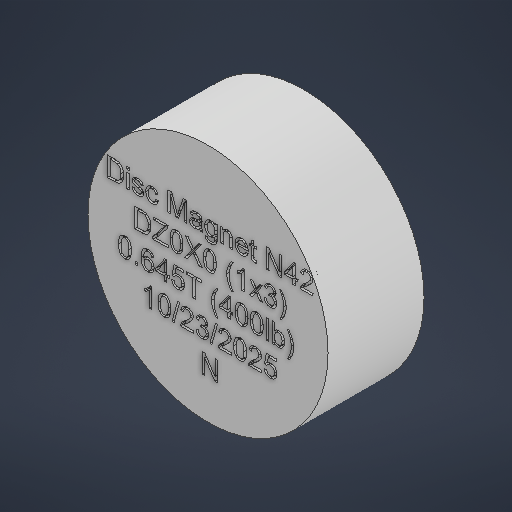
# Autodesk Inventor part: Sample_Magnet
Saved by Autodesk Inventor 2026.1 (Build 301233000, 233)
## iProperties
Created: 2025-10-23
Part Number: Sample_Magnet
Material: Generic
Document SubType Name: Modeling
Designer: usman
Density: 1 g/cm^3
Appearance: Default
Author: usman
Autodesk Inventor part; units mm, degrees
(part 1 of 2)
ref_plane "YZ Plane" through (0, 0, 0) normal (1, 0, 0) x (0, 1, 0)
ref_plane "XZ Plane" through (0, 0, 0) normal (0, 1, 0) x (-1, 0, 0)
ref_plane "XY Plane" through (0, 0, 0) normal (0, 0, 1) x (1, 0, 0)
sketch "Sketch1" plane through (0, 0, 0) normal (0, 0, 1) x (1, 0, 0)
  circle A0 centre (0, 0) radius 37.5
  dimension "d0" = 75
  constraints: 1 centre point, 1 coincident
  measures "d0" diameter of A0
extrude "Extrusion1" add sketch "Sketch1" along normal blind 30
sketch "Sketch2" plane through (0, 0, 30) normal (0, 0, 1) x (1, 0, 0)
  line L0 (-31.7477, 18.3387) -> (32.9347, 18.3387) construction
  line L1 (32.9347, 18.3387) -> (32.9347, -24.5034) construction
  line L2 (32.9347, -24.5034) -> (-31.7477, -24.5034) construction
  line L3 (-31.7477, -24.5034) -> (-31.7477, 18.3387) construction
  line L4 (-31.4082, 13.0446) -> (-31.4082, 19.1406)
  line L5 (-31.4082, 19.1406) -> (-29.308, 19.1406)
  spline S0 degree 2 poles (-29.308, 19.1406) (-28.5972, 19.1406) (-28.2208, 19.0523) knots 0 0 0 1 1 1
  spline S1 degree 2 poles (-28.2208, 19.0523) (-27.6958, 18.9315) (-27.3287, 18.6156) knots 0 0 0 1 1 1
  spline S2 degree 2 poles (-27.3287, 18.6156) (-26.8455, 18.2113) (-26.3669, 16.9429) (-26.3669, 16.1251) knots 0 0 0 1 2 2 2
  spline S3 degree 2 poles (-26.3669, 16.1251) (-26.3669, 15.4328) (-26.6922, 14.3595) (-27.1986, 13.6579) (-27.8026, 13.2537) (-28.6529, 13.0446) (-29.2058, 13.0446) knots 0 0 0 1 2 3 4 5 5 5
  line L6 (-29.2058, 13.0446) -> (-31.4082, 13.0446)
  line L7 (-30.5997, 13.7648) -> (-29.2988, 13.7648)
  spline S4 degree 2 poles (-29.2988, 13.7648) (-28.6947, 13.7648) (-28.0071, 13.9878) (-27.8073, 14.1922) knots 0 0 0 1 2 2 2
  spline S5 degree 2 poles (-27.8073, 14.1922) (-27.5192, 14.4803) (-27.1986, 15.4468) (-27.1986, 16.1391) knots 0 0 0 1 2 2 2
  spline S6 degree 2 poles (-27.1986, 16.1391) (-27.1986, 17.0962) (-27.8259, 18.123) (-28.2766, 18.295) knots 0 0 0 1 2 2 2
  spline S7 degree 2 poles (-28.2766, 18.295) (-28.6018, 18.4204) (-29.3173, 18.4204) knots 0 0 0 1 1 1
  line L8 (-29.3173, 18.4204) -> (-30.5997, 18.4204)
  line L9 (-30.5997, 18.4204) -> (-30.5997, 13.7648)
  line L10 (-25.3447, 13.0446) -> (-25.3447, 17.4633)
  line L11 (-25.3447, 17.4633) -> (-24.5967, 17.4633)
  line L12 (-24.5967, 17.4633) -> (-24.5967, 13.0446)
  line L13 (-24.5967, 13.0446) -> (-25.3447, 13.0446)
  line L14 (-25.3447, 18.281) -> (-25.3447, 19.1406)
  line L15 (-25.3447, 19.1406) -> (-24.5967, 19.1406)
  line L16 (-24.5967, 19.1406) -> (-24.5967, 18.281)
  line L17 (-24.5967, 18.281) -> (-25.3447, 18.281)
  line L18 (-23.7603, 14.3642) -> (-23.0215, 14.4803)
  spline S8 degree 2 poles (-23.0215, 14.4803) (-22.9611, 14.0343) (-22.3896, 13.5603) (-21.8739, 13.5603) knots 0 0 0 1 2 2 2
  spline S9 degree 2 poles (-21.8739, 13.5603) (-21.3582, 13.5603) (-20.8563, 13.9832) (-20.8563, 14.2666) knots 0 0 0 1 2 2 2
  spline S10 degree 2 poles (-20.8563, 14.2666) (-20.8563, 14.5175) (-21.0794, 14.6662) knots 0 0 0 1 1 1
  spline S11 degree 2 poles (-21.0794, 14.6662) (-21.2327, 14.7637) (-21.846, 14.9171) knots 0 0 0 1 1 1
  spline S12 degree 2 poles (-21.846, 14.9171) (-22.6684, 15.1262) (-23.305, 15.4282) (-23.6349, 15.9671) (-23.6349, 16.2877) knots 0 0 0 1 2 3 3 3
  spline S13 degree 2 poles (-23.6349, 16.2877) (-23.6349, 16.5851) (-23.3654, 17.0869) (-23.1331, 17.2542) knots 0 0 0 1 2 2 2
  spline S14 degree 2 poles (-23.1331, 17.2542) (-22.9565, 17.3843) (-22.3525, 17.5608) (-22.004, 17.5608) knots 0 0 0 1 2 2 2
  spline S15 degree 2 poles (-22.004, 17.5608) (-21.4836, 17.5608) (-20.6984, 17.2588) (-20.322, 16.7477) (-20.2523, 16.3203) knots 0 0 0 1 2 3 3 3
  line L19 (-20.2523, 16.3203) -> (-20.9864, 16.2227)
  spline S16 degree 2 poles (-20.9864, 16.2227) (-21.0376, 16.5665) (-21.5161, 16.9475) (-21.9529, 16.9475) knots 0 0 0 1 2 2 2
  spline S17 degree 2 poles (-21.9529, 16.9475) (-22.4686, 16.9475) (-22.91, 16.6037) (-22.91, 16.376) knots 0 0 0 1 2 2 2
  spline S18 degree 2 poles (-22.91, 16.376) (-22.91, 16.232) (-22.8171, 16.1158) knots 0 0 0 1 1 1
  spline S19 degree 2 poles (-22.8171, 16.1158) (-22.7288, 15.995) (-22.529, 15.916) knots 0 0 0 1 1 1
  spline S20 degree 2 poles (-22.529, 15.916) (-22.4175, 15.8742) (-21.8693, 15.7209) knots 0 0 0 1 1 1
  spline S21 degree 2 poles (-21.8693, 15.7209) (-21.0747, 15.5118) (-20.4428, 15.2423) (-20.0851, 14.7266) (-20.0851, 14.3409) knots 0 0 0 1 2 3 3 3
  spline S22 degree 2 poles (-20.0851, 14.3409) (-20.0851, 13.9692) (-20.5218, 13.3094) (-21.3489, 12.947) (-21.8693, 12.947) knots 0 0 0 1 2 3 3 3
  spline S23 degree 2 poles (-21.8693, 12.947) (-22.7288, 12.947) (-23.6349, 13.6626) (-23.7603, 14.3642) knots 0 0 0 1 2 2 2
  line L20 (-16.3122, 14.6615) -> (-15.5781, 14.564)
  spline S24 degree 2 poles (-15.5781, 14.564) (-15.6989, 13.8066) (-16.6932, 12.947) (-17.4181, 12.947) knots 0 0 0 1 2 2 2
  spline S25 degree 2 poles (-17.4181, 12.947) (-18.3241, 12.947) (-19.4253, 14.1318) (-19.4253, 15.2377) knots 0 0 0 1 2 2 2
  spline S26 degree 2 poles (-19.4253, 15.2377) (-19.4253, 15.9532) (-18.9513, 17.0265) (-17.9803, 17.5608) (-17.4134, 17.5608) knots 0 0 0 1 2 3 3 3
  spline S27 degree 2 poles (-17.4134, 17.5608) (-16.6932, 17.5608) (-15.7779, 16.8314) (-15.6478, 16.1623) knots 0 0 0 1 2 2 2
  line L21 (-15.6478, 16.1623) -> (-16.3773, 16.0508)
  spline S28 degree 2 poles (-16.3773, 16.0508) (-16.4795, 16.4968) (-17.0092, 16.9475) (-17.3809, 16.9475) knots 0 0 0 1 2 2 2
  spline S29 degree 2 poles (-17.3809, 16.9475) (-17.9477, 16.9475) (-18.654, 16.1344) (-18.654, 15.2563) knots 0 0 0 1 2 2 2
  spline S30 degree 2 poles (-18.654, 15.2563) (-18.654, 14.3688) (-17.971, 13.5603) (-17.4227, 13.5603) knots 0 0 0 1 2 2 2
  spline S31 degree 2 poles (-17.4227, 13.5603) (-16.9813, 13.5603) (-16.3912, 14.0993) (-16.3122, 14.6615) knots 0 0 0 1 2 2 2
  line L22 (-12.5022, 13.0446) -> (-12.5022, 19.1406)
  line L23 (-12.5022, 19.1406) -> (-11.2895, 19.1406)
  line L24 (-11.2895, 19.1406) -> (-9.8445, 14.8241)
  spline S32 degree 2 poles (-9.8445, 14.8241) (-9.6447, 14.2201) (-9.5518, 13.9228) knots 0 0 0 1 1 1
  spline S33 degree 2 poles (-9.5518, 13.9228) (-9.4496, 14.2526) (-9.2266, 14.8985) knots 0 0 0 1 1 1
  line L25 (-9.2266, 14.8985) -> (-7.763, 19.1406)
  line L26 (-7.763, 19.1406) -> (-6.6804, 19.1406)
  line L27 (-6.6804, 19.1406) -> (-6.6804, 13.0446)
  line L28 (-6.6804, 13.0446) -> (-7.4563, 13.0446)
  line L29 (-7.4563, 13.0446) -> (-7.4563, 18.1463)
  line L30 (-7.4563, 18.1463) -> (-9.2358, 13.0446)
  line L31 (-9.2358, 13.0446) -> (-9.9607, 13.0446)
  line L32 (-9.9607, 13.0446) -> (-11.7263, 18.2346)
  line L33 (-11.7263, 18.2346) -> (-11.7263, 13.0446)
  line L34 (-11.7263, 13.0446) -> (-12.5022, 13.0446)
  spline S34 degree 2 poles (-2.5962, 13.5882) (-3.0144, 13.2351) (-3.781, 12.947) (-4.2224, 12.947) knots 0 0 0 1 2 2 2
  spline S35 degree 2 poles (-4.2224, 12.947) (-4.9519, 12.947) (-5.7325, 13.6579) (-5.7325, 14.2108) knots 0 0 0 1 2 2 2
  spline S36 degree 2 poles (-5.7325, 14.2108) (-5.7325, 14.5361) (-5.4351, 15.0704) (-4.9612, 15.3956) (-4.6592, 15.4746) knots 0 0 0 1 2 3 3 3
  spline S37 degree 2 poles (-4.6592, 15.4746) (-4.4408, 15.535) (-3.9948, 15.5908) knots 0 0 0 1 1 1
  spline S38 degree 2 poles (-3.9948, 15.5908) (-3.0887, 15.6977) (-2.6613, 15.8463) knots 0 0 0 1 1 1
  spline S39 degree 2 poles (-2.6613, 15.8463) (-2.6566, 15.9997) (-2.6566, 16.0415) knots 0 0 0 1 1 1
  spline S40 degree 2 poles (-2.6566, 16.0415) (-2.6566, 16.5015) (-2.8704, 16.6873) knots 0 0 0 1 1 1
  spline S41 degree 2 poles (-2.8704, 16.6873) (-3.1538, 16.9429) (-3.7206, 16.9429) knots 0 0 0 1 1 1
  spline S42 degree 2 poles (-3.7206, 16.9429) (-4.2457, 16.9429) (-4.7475, 16.5712) (-4.8683, 16.1019) knots 0 0 0 1 2 2 2
  line L35 (-4.8683, 16.1019) -> (-5.6024, 16.1995)
  spline S43 degree 2 poles (-5.6024, 16.1995) (-5.5048, 16.6687) (-5.0448, 17.2495) (-4.1806, 17.5608) (-3.6138, 17.5608) knots 0 0 0 1 2 3 3 3
  spline S44 degree 2 poles (-3.6138, 17.5608) (-3.0469, 17.5608) (-2.3407, 17.296) (-2.0061, 16.8918) (-1.9411, 16.5851) knots 0 0 0 1 2 3 3 3
  spline S45 degree 2 poles (-1.9411, 16.5851) (-1.9039, 16.39) (-1.9039, 15.8928) knots 0 0 0 1 1 1
  line L36 (-1.9039, 15.8928) -> (-1.9039, 14.8938)
  spline S46 degree 2 poles (-1.9039, 14.8938) (-1.9039, 13.8531) (-1.8063, 13.3001) (-1.667, 13.0446) knots 0 0 0 1 2 2 2
  line L37 (-1.667, 13.0446) -> (-2.4475, 13.0446)
  spline S47 degree 2 poles (-2.4475, 13.0446) (-2.5637, 13.2769) (-2.5962, 13.5882) knots 0 0 0 1 1 1
  spline S48 degree 2 poles (-2.6566, 15.2609) (-3.0655, 15.0936) (-3.8786, 14.9775) knots 0 0 0 1 1 1
  spline S49 degree 2 poles (-3.8786, 14.9775) (-4.3433, 14.9124) (-4.7243, 14.7452) (-4.9333, 14.4246) (-4.9333, 14.2294) knots 0 0 0 1 2 3 3 3
  spline S50 degree 2 poles (-4.9333, 14.2294) (-4.9333, 13.932) (-4.4826, 13.5325) (-4.0459, 13.5325) knots 0 0 0 1 2 2 2
  spline S51 degree 2 poles (-4.0459, 13.5325) (-3.6138, 13.5325) (-2.9401, 13.9088) (-2.7821, 14.2387) knots 0 0 0 1 2 2 2
  spline S52 degree 2 poles (-2.7821, 14.2387) (-2.6613, 14.4943) (-2.6613, 14.9868) knots 0 0 0 1 1 1
  line L38 (-2.6613, 14.9868) -> (-2.6566, 15.2609)
  line L39 (-0.8817, 12.6822) -> (-0.1523, 12.5753)
  spline S53 degree 2 poles (-0.1523, 12.5753) (-0.1058, 12.2361) (0.1033, 12.0828) knots 0 0 0 1 1 1
  spline S54 degree 2 poles (0.1033, 12.0828) (0.3821, 11.8737) (0.8653, 11.8737) knots 0 0 0 1 1 1
  spline S55 degree 2 poles (0.8653, 11.8737) (1.381, 11.8737) (1.9479, 12.2872) (2.0501, 12.6636) knots 0 0 0 1 2 2 2
  spline S56 degree 2 poles (2.0501, 12.6636) (2.1059, 12.8913) (2.1012, 13.6207) knots 0 0 0 1 1 1
  spline S57 degree 2 poles (2.1012, 13.6207) (1.6134, 13.0446) (0.8792, 13.0446) knots 0 0 0 1 1 1
  spline S58 degree 2 poles (0.8792, 13.0446) (-0.0314, 13.0446) (-1.0304, 14.3595) (-1.0304, 15.2795) knots 0 0 0 1 2 2 2
  spline S59 degree 2 poles (-1.0304, 15.2795) (-1.0304, 15.9114) (-0.5704, 16.98) (0.2984, 17.5608) (0.8839, 17.5608) knots 0 0 0 1 2 3 3 3
  spline S60 degree 2 poles (0.8839, 17.5608) (1.6645, 17.5608) (2.1709, 16.9289) knots 0 0 0 1 1 1
  line L40 (2.1709, 16.9289) -> (2.1709, 17.4633)
  line L41 (2.1709, 17.4633) -> (2.8632, 17.4633)
  line L42 (2.8632, 17.4633) -> (2.8632, 13.6486)
  spline S61 degree 2 poles (2.8632, 13.6486) (2.8632, 12.6171) (2.4451, 11.7529) (1.5344, 11.2558) (0.8653, 11.2558) knots 0 0 0 1 2 3 3 3
  spline S62 degree 2 poles (0.8653, 11.2558) (0.0754, 11.2558) (-0.8957, 11.9666) (-0.8817, 12.6822) knots 0 0 0 1 2 2 2
  spline S63 degree 2 poles (-0.2591, 15.3306) (-0.2591, 14.4617) (0.4332, 13.6626) (0.9489, 13.6626) knots 0 0 0 1 2 2 2
  spline S64 degree 2 poles (0.9489, 13.6626) (1.4647, 13.6626) (2.1616, 14.4571) (2.1616, 15.3074) knots 0 0 0 1 2 2 2
  spline S65 degree 2 poles (2.1616, 15.3074) (2.1616, 16.1205) (1.4461, 16.9429) (0.9396, 16.9429) knots 0 0 0 1 2 2 2
  spline S66 degree 2 poles (0.9396, 16.9429) (0.4378, 16.9429) (-0.2591, 16.1298) (-0.2591, 15.3306) knots 0 0 0 1 2 2 2
  line L43 (3.9923, 13.0446) -> (3.9923, 17.4633)
  line L44 (3.9923, 17.4633) -> (4.666, 17.4633)
  line L45 (4.666, 17.4633) -> (4.666, 16.836)
  spline S67 degree 2 poles (4.666, 16.836) (5.1539, 17.5608) (6.0692, 17.5608) knots 0 0 0 1 1 1
  spline S68 degree 2 poles (6.0692, 17.5608) (6.4688, 17.5608) (7.1379, 17.2728) (7.4724, 16.8081) (7.5374, 16.4875) knots 0 0 0 1 2 3 3 3
  spline S69 degree 2 poles (7.5374, 16.4875) (7.5793, 16.2785) (7.5793, 15.7581) knots 0 0 0 1 1 1
  line L46 (7.5793, 15.7581) -> (7.5793, 13.0446)
  line L47 (7.5793, 13.0446) -> (6.8312, 13.0446)
  line L48 (6.8312, 13.0446) -> (6.8312, 15.7302)
  spline S70 degree 2 poles (6.8312, 15.7302) (6.8312, 16.1855) (6.6546, 16.6409) (6.2132, 16.9104) (5.9112, 16.9104) knots 0 0 0 1 2 3 3 3
  spline S71 degree 2 poles (5.9112, 16.9104) (5.4327, 16.9104) (4.7403, 16.3017) (4.7403, 15.456) knots 0 0 0 1 2 2 2
  line L49 (4.7403, 15.456) -> (4.7403, 13.0446)
  line L50 (4.7403, 13.0446) -> (3.9923, 13.0446)
  line L51 (11.747, 14.471) -> (12.523, 14.3735)
  spline S72 degree 2 poles (12.523, 14.3735) (12.3371, 13.6951) (11.3474, 12.947) (10.5808, 12.947) knots 0 0 0 1 2 2 2
  spline S73 degree 2 poles (10.5808, 12.947) (9.6097, 12.947) (8.476, 14.1411) (8.476, 15.2144) knots 0 0 0 1 2 2 2
  spline S74 degree 2 poles (8.476, 15.2144) (8.476, 16.3296) (9.6237, 17.5608) (10.539, 17.5608) knots 0 0 0 1 2 2 2
  spline S75 degree 2 poles (10.539, 17.5608) (11.4218, 17.5608) (12.5462, 16.3528) (12.5462, 15.2609) knots 0 0 0 1 2 2 2
  spline S76 degree 2 poles (12.5462, 15.2609) (12.5462, 15.1959) (12.5416, 15.0611) knots 0 0 0 1 1 1
  line L52 (12.5416, 15.0611) -> (9.2473, 15.0611)
  spline S77 degree 2 poles (9.2473, 15.0611) (9.2891, 14.3316) (10.0279, 13.5603) (10.5808, 13.5603) knots 0 0 0 1 2 2 2
  spline S78 degree 2 poles (10.5808, 13.5603) (10.9943, 13.5603) (11.5751, 13.9971) (11.747, 14.471) knots 0 0 0 1 2 2 2
  line L53 (9.2891, 15.6744) -> (11.7563, 15.6744)
  spline S79 degree 2 poles (11.7563, 15.6744) (11.7052, 16.232) (11.4729, 16.5154) knots 0 0 0 1 1 1
  spline S80 degree 2 poles (11.4729, 16.5154) (11.1151, 16.9475) (10.5436, 16.9475) knots 0 0 0 1 1 1
  spline S81 degree 2 poles (10.5436, 16.9475) (10.0279, 16.9475) (9.3263, 16.2552) (9.2891, 15.6744) knots 0 0 0 1 2 2 2
  line L54 (15.0924, 13.7137) -> (15.1993, 13.0492)
  spline S82 degree 2 poles (15.1993, 13.0492) (14.8833, 12.9842) (14.6324, 12.9842) knots 0 0 0 1 1 1
  spline S83 degree 2 poles (14.6324, 12.9842) (14.2282, 12.9842) (13.7775, 13.2444) (13.5963, 13.6626) (13.5963, 14.3363) knots 0 0 0 1 2 3 3 3
  line L55 (13.5963, 14.3363) -> (13.5963, 16.8825)
  line L56 (13.5963, 16.8825) -> (13.0434, 16.8825)
  line L57 (13.0434, 16.8825) -> (13.0434, 17.4633)
  line L58 (13.0434, 17.4633) -> (13.5963, 17.4633)
  line L59 (13.5963, 17.4633) -> (13.5963, 18.5552)
  line L60 (13.5963, 18.5552) -> (14.3443, 19.0059)
  line L61 (14.3443, 19.0059) -> (14.3443, 17.4633)
  line L62 (14.3443, 17.4633) -> (15.0924, 17.4633)
  line L63 (15.0924, 17.4633) -> (15.0924, 16.8825)
  line L64 (15.0924, 16.8825) -> (14.3443, 16.8825)
  line L65 (14.3443, 16.8825) -> (14.3443, 14.2945)
  spline S84 degree 2 poles (14.3443, 14.2945) (14.3443, 13.9739) (14.4233, 13.788) (14.5999, 13.6811) (14.7672, 13.6811) knots 0 0 0 1 2 3 3 3
  spline S85 degree 2 poles (14.7672, 13.6811) (14.888, 13.6811) (15.0924, 13.7137) knots 0 0 0 1 1 1
  line L66 (18.2798, 13.0446) -> (18.2798, 19.1406)
  line L67 (18.2798, 19.1406) -> (19.1068, 19.1406)
  line L68 (19.1068, 19.1406) -> (22.3128, 14.3549)
  line L69 (22.3128, 14.3549) -> (22.3128, 19.1406)
  line L70 (22.3128, 19.1406) -> (23.0841, 19.1406)
  line L71 (23.0841, 19.1406) -> (23.0841, 13.0446)
  line L72 (23.0841, 13.0446) -> (22.2571, 13.0446)
  line L73 (22.2571, 13.0446) -> (19.0511, 17.8303)
  line L74 (19.0511, 17.8303) -> (19.0511, 13.0446)
  line L75 (19.0511, 13.0446) -> (18.2798, 13.0446)
  line L76 (26.5317, 13.0446) -> (26.5317, 14.5035)
  line L77 (26.5317, 14.5035) -> (23.8879, 14.5035)
  line L78 (23.8879, 14.5035) -> (23.8879, 15.1912)
  line L79 (23.8879, 15.1912) -> (26.6664, 19.1406)
  line L80 (26.6664, 19.1406) -> (27.2797, 19.1406)
  line L81 (27.2797, 19.1406) -> (27.2797, 15.1912)
  line L82 (27.2797, 15.1912) -> (28.1022, 15.1912)
  line L83 (28.1022, 15.1912) -> (28.1022, 14.5035)
  line L84 (28.1022, 14.5035) -> (27.2797, 14.5035)
  line L85 (27.2797, 14.5035) -> (27.2797, 13.0446)
  line L86 (27.2797, 13.0446) -> (26.5317, 13.0446)
  line L87 (26.5317, 15.1912) -> (26.5317, 17.9418)
  line L88 (26.5317, 17.9418) -> (24.622, 15.1912)
  line L89 (24.622, 15.1912) -> (26.5317, 15.1912)
  line L90 (32.7996, 13.7648) -> (32.7996, 13.0446)
  line L91 (32.7996, 13.0446) -> (28.7712, 13.0446)
  spline S86 degree 2 poles (28.7712, 13.0446) (28.7619, 13.3141) (28.8595, 13.565) knots 0 0 0 1 1 1
  spline S87 degree 2 poles (28.8595, 13.565) (29.0128, 13.9785) (29.6912, 14.773) (30.3324, 15.2981) knots 0 0 0 1 2 2 2
  spline S88 degree 2 poles (30.3324, 15.2981) (31.3221, 16.1158) (32.019, 17.0637) (32.019, 17.4911) knots 0 0 0 1 2 2 2
  spline S89 degree 2 poles (32.019, 17.4911) (32.019, 17.9372) (31.3825, 18.5459) (30.8714, 18.5459) knots 0 0 0 1 2 2 2
  spline S90 degree 2 poles (30.8714, 18.5459) (30.3324, 18.5459) (29.6866, 17.8954) (29.6819, 17.3239) knots 0 0 0 1 2 2 2
  line L92 (29.6819, 17.3239) -> (28.9106, 17.4029)
  spline S91 degree 2 poles (28.9106, 17.4029) (28.9896, 18.2624) (30.0211, 19.1638) (30.89, 19.1638) knots 0 0 0 1 2 2 2
  spline S92 degree 2 poles (30.89, 19.1638) (31.7681, 19.1638) (32.7903, 18.1927) (32.7903, 17.4726) knots 0 0 0 1 2 2 2
  spline S93 degree 2 poles (32.7903, 17.4726) (32.7903, 17.1055) (32.4929, 16.3993) (31.796, 15.6187) (30.9922, 14.9357) knots 0 0 0 1 2 3 3 3
  spline S94 degree 2 poles (30.9922, 14.9357) (30.3185, 14.3735) (29.9375, 13.9692) (29.812, 13.7648) knots 0 0 0 1 2 2 2
  line L93 (29.812, 13.7648) -> (32.7996, 13.7648)
  line L94 (-22.8868, 3.4513) -> (-22.8868, 9.5473)
  line L95 (-22.8868, 9.5473) -> (-20.7867, 9.5473)
  spline S95 degree 2 poles (-20.7867, 9.5473) (-20.0758, 9.5473) (-19.6994, 9.459) knots 0 0 0 1 1 1
  spline S96 degree 2 poles (-19.6994, 9.459) (-19.1744, 9.3382) (-18.8073, 9.0223) knots 0 0 0 1 1 1
  spline S97 degree 2 poles (-18.8073, 9.0223) (-18.3241, 8.618) (-17.8455, 7.3496) (-17.8455, 6.5318) knots 0 0 0 1 2 2 2
  spline S98 degree 2 poles (-17.8455, 6.5318) (-17.8455, 5.8395) (-18.1708, 4.7662) (-18.6772, 4.0646) (-19.2812, 3.6604) (-20.1315, 3.4513) (-20.6844, 3.4513) knots 0 0 0 1 2 3 4 5 5 5
  line L96 (-20.6844, 3.4513) -> (-22.8868, 3.4513)
  line L97 (-22.0783, 4.1715) -> (-20.7774, 4.1715)
  spline S99 degree 2 poles (-20.7774, 4.1715) (-20.1733, 4.1715) (-19.4857, 4.3945) (-19.2859, 4.599) knots 0 0 0 1 2 2 2
  spline S100 degree 2 poles (-19.2859, 4.599) (-18.9978, 4.887) (-18.6772, 5.8535) (-18.6772, 6.5458) knots 0 0 0 1 2 2 2
  spline S101 degree 2 poles (-18.6772, 6.5458) (-18.6772, 7.5029) (-19.3045, 8.5298) (-19.7552, 8.7017) knots 0 0 0 1 2 2 2
  spline S102 degree 2 poles (-19.7552, 8.7017) (-20.0804, 8.8271) (-20.7959, 8.8271) knots 0 0 0 1 1 1
  line L98 (-20.7959, 8.8271) -> (-22.0783, 8.8271)
  line L99 (-22.0783, 8.8271) -> (-22.0783, 4.1715)
  line L100 (-17.2229, 3.4513) -> (-17.2229, 4.1994)
  line L101 (-17.2229, 4.1994) -> (-14.0959, 8.1023)
  spline S103 degree 2 poles (-14.0959, 8.1023) (-13.7614, 8.5158) (-13.4594, 8.8271) knots 0 0 0 1 1 1
  line L102 (-13.4594, 8.8271) -> (-16.8698, 8.8271)
  line L103 (-16.8698, 8.8271) -> (-16.8698, 9.5473)
  line L104 (-16.8698, 9.5473) -> (-12.4976, 9.5473)
  line L105 (-12.4976, 9.5473) -> (-12.4976, 8.8271)
  line L106 (-12.4976, 8.8271) -> (-15.9266, 4.6036)
  line L107 (-15.9266, 4.6036) -> (-16.2936, 4.1715)
  line L108 (-16.2936, 4.1715) -> (-12.4, 4.1715)
  line L109 (-12.4, 4.1715) -> (-12.4, 3.4513)
  line L110 (-12.4, 3.4513) -> (-17.2229, 3.4513)
  spline S104 degree 2 poles (-11.8332, 6.4575) (-11.8332, 7.5401) (-11.3871, 8.8596) (-10.5136, 9.5705) (-9.8445, 9.5705) knots 0 0 0 1 2 3 3 3
  spline S105 degree 2 poles (-9.8445, 9.5705) (-9.3567, 9.5705) (-8.6132, 9.1756) (-8.1347, 8.4322) (-7.8605, 7.3635) (-7.8605, 6.4575) knots 0 0 0 1 2 3 4 4 4
  spline S106 degree 2 poles (-7.8605, 6.4575) (-7.8605, 5.3842) (-8.3019, 4.0646) (-9.1801, 3.3491) (-9.8445, 3.3491) knots 0 0 0 1 2 3 3 3
  spline S107 degree 2 poles (-9.8445, 3.3491) (-10.7273, 3.3491) (-11.2291, 3.9763) knots 0 0 0 1 1 1
  spline S108 degree 2 poles (-11.2291, 3.9763) (-11.8332, 4.743) (-11.8332, 6.4575) knots 0 0 0 1 1 1
  spline S109 degree 2 poles (-11.0619, 6.4575) (-11.0619, 4.9521) (-10.3603, 3.9624) (-9.8445, 3.9624) knots 0 0 0 1 2 2 2
  spline S110 degree 2 poles (-9.8445, 3.9624) (-9.3334, 3.9624) (-8.6318, 4.9567) (-8.6318, 6.4575) knots 0 0 0 1 2 2 2
  spline S111 degree 2 poles (-8.6318, 6.4575) (-8.6318, 7.9629) (-9.3334, 8.9526) (-9.8538, 8.9526) knots 0 0 0 1 2 2 2
  spline S112 degree 2 poles (-9.8538, 8.9526) (-10.3696, 8.9526) (-10.6762, 8.5158) knots 0 0 0 1 1 1
  spline S113 degree 2 poles (-10.6762, 8.5158) (-11.0619, 7.9583) (-11.0619, 6.4575) knots 0 0 0 1 1 1
  line L111 (-7.4145, 3.4513) -> (-5.0588, 6.6108)
  line L112 (-5.0588, 6.6108) -> (-7.1357, 9.5473)
  line L113 (-7.1357, 9.5473) -> (-6.1786, 9.5473)
  line L114 (-6.1786, 9.5473) -> (-5.0634, 7.9861)
  spline S114 degree 2 poles (-5.0634, 7.9861) (-4.715, 7.5029) (-4.5756, 7.2381) knots 0 0 0 1 1 1
  spline S115 degree 2 poles (-4.5756, 7.2381) (-4.3711, 7.5633) (-4.0877, 7.9257) knots 0 0 0 1 1 1
  line L115 (-4.0877, 7.9257) -> (-2.8704, 9.5473)
  line L116 (-2.8704, 9.5473) -> (-1.9922, 9.5473)
  line L117 (-1.9922, 9.5473) -> (-4.1063, 6.648)
  line L118 (-4.1063, 6.648) -> (-1.8249, 3.4513)
  line L119 (-1.8249, 3.4513) -> (-2.8146, 3.4513)
  line L120 (-2.8146, 3.4513) -> (-4.3572, 5.6258)
  spline S116 degree 2 poles (-4.3572, 5.6258) (-4.4873, 5.8116) (-4.6127, 6.0021) knots 0 0 0 1 1 1
  spline S117 degree 2 poles (-4.6127, 6.0021) (-4.8125, 5.6908) (-4.9008, 5.5654) knots 0 0 0 1 1 1
  line L121 (-4.9008, 5.5654) -> (-6.4434, 3.4513)
  line L122 (-6.4434, 3.4513) -> (-7.4145, 3.4513)
  spline S118 degree 2 poles (-1.4161, 6.4575) (-1.4161, 7.5401) (-0.97, 8.8596) (-0.0965, 9.5705) (0.5726, 9.5705) knots 0 0 0 1 2 3 3 3
  spline S119 degree 2 poles (0.5726, 9.5705) (1.0604, 9.5705) (1.8039, 9.1756) (2.2824, 8.4322) (2.5566, 7.3635) (2.5566, 6.4575) knots 0 0 0 1 2 3 4 4 4
  spline S120 degree 2 poles (2.5566, 6.4575) (2.5566, 5.3842) (2.1152, 4.0646) (1.237, 3.3491) (0.5726, 3.3491) knots 0 0 0 1 2 3 3 3
  spline S121 degree 2 poles (0.5726, 3.3491) (-0.3102, 3.3491) (-0.812, 3.9763) knots 0 0 0 1 1 1
  spline S122 degree 2 poles (-0.812, 3.9763) (-1.4161, 4.743) (-1.4161, 6.4575) knots 0 0 0 1 1 1
  spline S123 degree 2 poles (-0.6448, 6.4575) (-0.6448, 4.9521) (0.0568, 3.9624) (0.5726, 3.9624) knots 0 0 0 1 2 2 2
  spline S124 degree 2 poles (0.5726, 3.9624) (1.0837, 3.9624) (1.7853, 4.9567) (1.7853, 6.4575) knots 0 0 0 1 2 2 2
  spline S125 degree 2 poles (1.7853, 6.4575) (1.7853, 7.9629) (1.0837, 8.9526) (0.5633, 8.9526) knots 0 0 0 1 2 2 2
  spline S126 degree 2 poles (0.5633, 8.9526) (0.0475, 8.9526) (-0.2591, 8.5158) knots 0 0 0 1 1 1
  spline S127 degree 2 poles (-0.2591, 8.5158) (-0.6448, 7.9583) (-0.6448, 6.4575) knots 0 0 0 1 1 1
  spline S128 degree 2 poles (7.3237, 1.6578) (6.7058, 2.4384) (5.8462, 4.5339) (5.8462, 5.6583) knots 0 0 0 1 2 2 2
  spline S129 degree 2 poles (5.8462, 5.6583) (5.8462, 6.648) (6.1668, 7.554) knots 0 0 0 1 1 1
  spline S130 degree 2 poles (6.1668, 7.554) (6.5431, 8.6041) (7.3237, 9.6495) knots 0 0 0 1 1 1
  line L123 (7.3237, 9.6495) -> (7.858, 9.6495)
  spline S131 degree 2 poles (7.858, 9.6495) (7.3562, 8.7853) (7.1936, 8.4136) knots 0 0 0 1 1 1
  spline S132 degree 2 poles (7.1936, 8.4136) (6.9427, 7.8421) (6.794, 7.2148) knots 0 0 0 1 1 1
  spline S133 degree 2 poles (6.794, 7.2148) (6.6175, 6.4389) (6.6175, 5.6537) knots 0 0 0 1 1 1
  spline S134 degree 2 poles (6.6175, 5.6537) (6.6175, 3.6557) (7.858, 1.6578) knots 0 0 0 1 1 1
  line L124 (7.858, 1.6578) -> (7.3237, 1.6578)
  line L125 (11.3335, 3.4513) -> (10.5854, 3.4513)
  line L126 (10.5854, 3.4513) -> (10.5854, 8.2185)
  spline S135 degree 2 poles (10.5854, 8.2185) (10.316, 7.9629) (9.4378, 7.4472) (9.0893, 7.3171) knots 0 0 0 1 2 2 2
  line L127 (9.0893, 7.3171) -> (9.0893, 8.0419)
  spline S136 degree 2 poles (9.0893, 8.0419) (9.7166, 8.3346) (10.6551, 9.1756) (10.8503, 9.5705) knots 0 0 0 1 2 2 2
  line L128 (10.8503, 9.5705) -> (11.3335, 9.5705)
  line L129 (11.3335, 9.5705) -> (11.3335, 3.4513)
  line L130 (12.9597, 3.4513) -> (14.5767, 5.7373)
  line L131 (14.5767, 5.7373) -> (13.0805, 7.87)
  line L132 (13.0805, 7.87) -> (14.0098, 7.87)
  line L133 (14.0098, 7.87) -> (14.6975, 6.8338)
  spline S137 degree 2 poles (14.6975, 6.8338) (14.8926, 6.5411) (15.0088, 6.346) knots 0 0 0 1 1 1
  spline S138 degree 2 poles (15.0088, 6.346) (15.1946, 6.6062) (15.3433, 6.8199) knots 0 0 0 1 1 1
  line L134 (15.3433, 6.8199) -> (16.0867, 7.87)
  line L135 (16.0867, 7.87) -> (16.9881, 7.87)
  line L136 (16.9881, 7.87) -> (15.492, 5.7512)
  line L137 (15.492, 5.7512) -> (17.095, 3.4513)
  line L138 (17.095, 3.4513) -> (16.175, 3.4513)
  line L139 (16.175, 3.4513) -> (15.2643, 4.8173)
  line L140 (15.2643, 4.8173) -> (15.0506, 5.1519)
  line L141 (15.0506, 5.1519) -> (13.8658, 3.4513)
  line L142 (13.8658, 3.4513) -> (12.9597, 3.4513)
  line L143 (17.5178, 5.0682) -> (18.2658, 5.1658)
  spline S139 degree 2 poles (18.2658, 5.1658) (18.3959, 4.5293) (19.0139, 3.9671) (19.46, 3.9671) knots 0 0 0 1 2 2 2
  spline S140 degree 2 poles (19.46, 3.9671) (19.9896, 3.9671) (20.7145, 4.7012) (20.7145, 5.2401) knots 0 0 0 1 2 2 2
  spline S141 degree 2 poles (20.7145, 5.2401) (20.7145, 5.7559) (20.0408, 6.425) (19.5204, 6.425) knots 0 0 0 1 2 2 2
  spline S142 degree 2 poles (19.5204, 6.425) (19.3113, 6.425) (18.9953, 6.3413) knots 0 0 0 1 1 1
  line L144 (18.9953, 6.3413) -> (19.0743, 6.9965)
  spline S143 degree 2 poles (19.0743, 6.9965) (19.1533, 6.9872) (19.1951, 6.9872) knots 0 0 0 1 1 1
  spline S144 degree 2 poles (19.1951, 6.9872) (19.6737, 6.9872) (20.4403, 7.489) (20.4403, 8.0047) knots 0 0 0 1 2 2 2
  spline S145 degree 2 poles (20.4403, 8.0047) (20.4403, 8.4182) (19.8828, 8.9572) (19.4414, 8.9572) knots 0 0 0 1 2 2 2
  spline S146 degree 2 poles (19.4414, 8.9572) (19.0046, 8.9572) (18.4238, 8.409) (18.3402, 7.856) knots 0 0 0 1 2 2 2
  line L145 (18.3402, 7.856) -> (17.5921, 7.9908)
  spline S147 degree 2 poles (17.5921, 7.9908) (17.7315, 8.7435) (18.7026, 9.5705) (19.4274, 9.5705) knots 0 0 0 1 2 2 2
  spline S148 degree 2 poles (19.4274, 9.5705) (19.9246, 9.5705) (20.7656, 9.1431) (21.2116, 8.4043) (21.2116, 7.9908) knots 0 0 0 1 2 3 3 3
  spline S149 degree 2 poles (21.2116, 7.9908) (21.2116, 7.5958) (20.7888, 6.9454) (20.3706, 6.7549) knots 0 0 0 1 2 2 2
  spline S150 degree 2 poles (20.3706, 6.7549) (20.9143, 6.6294) (21.509, 5.8442) (21.509, 5.2541) knots 0 0 0 1 2 2 2
  spline S151 degree 2 poles (21.509, 5.2541) (21.509, 4.4596) (20.3428, 3.3491) (19.4553, 3.3491) knots 0 0 0 1 2 2 2
  spline S152 degree 2 poles (19.4553, 3.3491) (18.6515, 3.3491) (17.5921, 4.3062) (17.5178, 5.0682) knots 0 0 0 1 2 2 2
  line L146 (22.9447, 1.6578) -> (22.4104, 1.6578)
  spline S153 degree 2 poles (22.4104, 1.6578) (23.651, 3.6557) (23.651, 5.6537) knots 0 0 0 1 1 1
  spline S154 degree 2 poles (23.651, 5.6537) (23.651, 6.4343) (23.4744, 7.2056) knots 0 0 0 1 1 1
  spline S155 degree 2 poles (23.4744, 7.2056) (23.3304, 7.8282) (23.0795, 8.4043) knots 0 0 0 1 1 1
  spline S156 degree 2 poles (23.0795, 8.4043) (22.9168, 8.776) (22.4104, 9.6495) knots 0 0 0 1 1 1
  line L147 (22.4104, 9.6495) -> (22.9447, 9.6495)
  spline S157 degree 2 poles (22.9447, 9.6495) (23.7253, 8.6041) (24.1017, 7.554) knots 0 0 0 1 1 1
  spline S158 degree 2 poles (24.1017, 7.554) (24.4223, 6.648) (24.4223, 5.6583) knots 0 0 0 1 1 1
  spline S159 degree 2 poles (24.4223, 5.6583) (24.4223, 4.5339) (23.5627, 2.4384) (22.9447, 1.6578) knots 0 0 0 1 2 2 2
  spline S160 degree 2 poles (-27.9211, -3.1358) (-27.9211, -2.0532) (-27.4751, -0.7336) (-26.6015, -0.0228) (-25.9325, -0.0228) knots 0 0 0 1 2 3 3 3
  spline S161 degree 2 poles (-25.9325, -0.0228) (-25.4446, -0.0228) (-24.7012, -0.4177) (-24.2226, -1.1611) (-23.9485, -2.2298) (-23.9485, -3.1358) knots 0 0 0 1 2 3 4 4 4
  spline S162 degree 2 poles (-23.9485, -3.1358) (-23.9485, -4.2091) (-24.3899, -5.5287) (-25.268, -6.2442) (-25.9325, -6.2442) knots 0 0 0 1 2 3 3 3
  spline S163 degree 2 poles (-25.9325, -6.2442) (-26.8153, -6.2442) (-27.3171, -5.6169) knots 0 0 0 1 1 1
  spline S164 degree 2 poles (-27.3171, -5.6169) (-27.9211, -4.8503) (-27.9211, -3.1358) knots 0 0 0 1 1 1
  spline S165 degree 2 poles (-27.1498, -3.1358) (-27.1498, -4.6412) (-26.4482, -5.6309) (-25.9325, -5.6309) knots 0 0 0 1 2 2 2
  spline S166 degree 2 poles (-25.9325, -5.6309) (-25.4214, -5.6309) (-24.7198, -4.6366) (-24.7198, -3.1358) knots 0 0 0 1 2 2 2
  spline S167 degree 2 poles (-24.7198, -3.1358) (-24.7198, -1.6304) (-25.4214, -0.6407) (-25.9418, -0.6407) knots 0 0 0 1 2 2 2
  spline S168 degree 2 poles (-25.9418, -0.6407) (-26.4575, -0.6407) (-26.7642, -1.0775) knots 0 0 0 1 1 1
  spline S169 degree 2 poles (-26.7642, -1.0775) (-27.1498, -1.635) (-27.1498, -3.1358) knots 0 0 0 1 1 1
  line L148 (-22.7683, -6.142) -> (-22.7683, -5.2917)
  line L149 (-22.7683, -5.2917) -> (-21.918, -5.2917)
  line L150 (-21.918, -5.2917) -> (-21.918, -6.142)
  line L151 (-21.918, -6.142) -> (-22.7683, -6.142)
  line L152 (-16.9325, -1.5421) -> (-17.6759, -1.6025)
  spline S170 degree 2 poles (-17.6759, -1.6025) (-17.7781, -1.1611) (-17.9594, -0.9567) knots 0 0 0 1 1 1
  spline S171 degree 2 poles (-17.9594, -0.9567) (-18.266, -0.6361) (-18.7121, -0.6361) knots 0 0 0 1 1 1
  spline S172 degree 2 poles (-18.7121, -0.6361) (-19.0698, -0.6361) (-19.3393, -0.8359) knots 0 0 0 1 1 1
  spline S173 degree 2 poles (-19.3393, -0.8359) (-19.6924, -1.0914) (-20.1013, -2.0857) (-20.1106, -3.0011) knots 0 0 0 1 2 2 2
  spline S174 degree 2 poles (-20.1106, -3.0011) (-19.8411, -2.5875) (-19.0559, -2.1879) (-18.6284, -2.1879) knots 0 0 0 1 2 2 2
  spline S175 degree 2 poles (-18.6284, -2.1879) (-17.8804, -2.1879) (-16.8256, -3.2891) (-16.8256, -4.1626) knots 0 0 0 1 2 2 2
  spline S176 degree 2 poles (-16.8256, -4.1626) (-16.8256, -4.7341) (-17.3228, -5.7192) (-18.187, -6.2442) (-18.7353, -6.2442) knots 0 0 0 1 2 3 3 3
  spline S177 degree 2 poles (-18.7353, -6.2442) (-19.6739, -6.2442) (-20.854, -4.8689) (-20.854, -3.2891) knots 0 0 0 1 2 2 2
  spline S178 degree 2 poles (-20.854, -3.2891) (-20.854, -1.5235) (-20.1989, -0.7197) knots 0 0 0 1 1 1
  spline S179 degree 2 poles (-20.1989, -0.7197) (-19.632, -0.0228) (-18.6656, -0.0228) knots 0 0 0 1 1 1
  spline S180 degree 2 poles (-18.6656, -0.0228) (-17.9454, -0.0228) (-17.0254, -0.8312) (-16.9325, -1.5421) knots 0 0 0 1 2 2 2
  spline S181 degree 2 poles (-19.9945, -4.1673) (-19.9945, -4.5529) (-19.6646, -5.2592) (-19.0791, -5.6309) (-18.7539, -5.6309) knots 0 0 0 1 2 3 3 3
  spline S182 degree 2 poles (-18.7539, -5.6309) (-18.2753, -5.6309) (-17.5969, -4.8642) (-17.5969, -4.2091) knots 0 0 0 1 2 2 2
  spline S183 degree 2 poles (-17.5969, -4.2091) (-17.5969, -3.5772) (-18.266, -2.8477) (-18.7818, -2.8477) knots 0 0 0 1 2 2 2
  spline S184 degree 2 poles (-18.7818, -2.8477) (-19.2882, -2.8477) (-19.9945, -3.5772) (-19.9945, -4.1673) knots 0 0 0 1 2 2 2
  line L153 (-13.6894, -6.142) -> (-13.6894, -4.683)
  line L154 (-13.6894, -4.683) -> (-16.3331, -4.683)
  line L155 (-16.3331, -4.683) -> (-16.3331, -3.9954)
  line L156 (-16.3331, -3.9954) -> (-13.5546, -0.046)
  line L157 (-13.5546, -0.046) -> (-12.9413, -0.046)
  line L158 (-12.9413, -0.046) -> (-12.9413, -3.9954)
  line L159 (-12.9413, -3.9954) -> (-12.1189, -3.9954)
  line L160 (-12.1189, -3.9954) -> (-12.1189, -4.683)
  line L161 (-12.1189, -4.683) -> (-12.9413, -4.683)
  line L162 (-12.9413, -4.683) -> (-12.9413, -6.142)
  line L163 (-12.9413, -6.142) -> (-13.6894, -6.142)
  line L164 (-13.6894, -3.9954) -> (-13.6894, -1.2447)
  line L165 (-13.6894, -1.2447) -> (-15.599, -3.9954)
  line L166 (-15.599, -3.9954) -> (-13.6894, -3.9954)
  line L167 (-11.3523, -4.5436) -> (-10.567, -4.4786)
  spline S185 degree 2 poles (-10.567, -4.4786) (-10.4787, -5.0547) (-9.8468, -5.6309) (-9.3961, -5.6309) knots 0 0 0 1 2 2 2
  spline S186 degree 2 poles (-9.3961, -5.6309) (-8.8479, -5.6309) (-8.1045, -4.8131) (-8.1045, -4.1394) knots 0 0 0 1 2 2 2
  spline S187 degree 2 poles (-8.1045, -4.1394) (-8.1045, -3.4982) (-8.82, -2.7548) (-9.4054, -2.7548) knots 0 0 0 1 2 2 2
  spline S188 degree 2 poles (-9.4054, -2.7548) (-9.7679, -2.7548) (-10.3486, -3.0847) (-10.5159, -3.3495) knots 0 0 0 1 2 2 2
  line L168 (-10.5159, -3.3495) -> (-11.2175, -3.2566)
  line L169 (-11.2175, -3.2566) -> (-10.6274, -0.125)
  line L170 (-10.6274, -0.125) -> (-7.598, -0.125)
  line L171 (-7.598, -0.125) -> (-7.598, -0.8405)
  line L172 (-7.598, -0.8405) -> (-10.028, -0.8405)
  line L173 (-10.028, -0.8405) -> (-10.3579, -2.476)
  spline S189 degree 2 poles (-10.3579, -2.476) (-9.8097, -2.095) (-9.2056, -2.095) knots 0 0 0 1 1 1
  spline S190 degree 2 poles (-9.2056, -2.095) (-8.4065, -2.095) (-7.3099, -3.2008) (-7.3099, -4.0697) knots 0 0 0 1 2 2 2
  spline S191 degree 2 poles (-7.3099, -4.0697) (-7.3099, -4.9014) (-7.7932, -5.5054) knots 0 0 0 1 1 1
  spline S192 degree 2 poles (-7.7932, -5.5054) (-8.3786, -6.2442) (-9.3915, -6.2442) knots 0 0 0 1 1 1
  spline S193 degree 2 poles (-9.3915, -6.2442) (-10.2232, -6.2442) (-11.2779, -5.3149) (-11.3523, -4.5436) knots 0 0 0 1 2 2 2
  line L174 (-4.7637, -6.142) -> (-4.7637, -0.7662)
  line L175 (-4.7637, -0.7662) -> (-6.771, -0.7662)
  line L176 (-6.771, -0.7662) -> (-6.771, -0.046)
  line L177 (-6.771, -0.046) -> (-1.9388, -0.046)
  line L178 (-1.9388, -0.046) -> (-1.9388, -0.7662)
  line L179 (-1.9388, -0.7662) -> (-3.9553, -0.7662)
  line L180 (-3.9553, -0.7662) -> (-3.9553, -6.142)
  line L181 (-3.9553, -6.142) -> (-4.7637, -6.142)
  spline S194 degree 2 poles (2.5914, -7.9355) (1.9735, -7.1549) (1.1139, -5.0594) (1.1139, -3.935) knots 0 0 0 1 2 2 2
  spline S195 degree 2 poles (1.1139, -3.935) (1.1139, -2.9453) (1.4345, -2.0393) knots 0 0 0 1 1 1
  spline S196 degree 2 poles (1.4345, -2.0393) (1.8108, -0.9892) (2.5914, 0.0562) knots 0 0 0 1 1 1
  line L182 (2.5914, 0.0562) -> (3.1257, 0.0562)
  spline S197 degree 2 poles (3.1257, 0.0562) (2.6239, -0.808) (2.4613, -1.1797) knots 0 0 0 1 1 1
  spline S198 degree 2 poles (2.4613, -1.1797) (2.2104, -1.7512) (2.0617, -2.3784) knots 0 0 0 1 1 1
  spline S199 degree 2 poles (2.0617, -2.3784) (1.8852, -3.1544) (1.8852, -3.9396) knots 0 0 0 1 1 1
  spline S200 degree 2 poles (1.8852, -3.9396) (1.8852, -5.9375) (3.1257, -7.9355) knots 0 0 0 1 1 1
  line L183 (3.1257, -7.9355) -> (2.5914, -7.9355)
  line L184 (6.183, -6.142) -> (6.183, -4.683)
  line L185 (6.183, -4.683) -> (3.5393, -4.683)
  line L186 (3.5393, -4.683) -> (3.5393, -3.9954)
  line L187 (3.5393, -3.9954) -> (6.3178, -0.046)
  line L188 (6.3178, -0.046) -> (6.9311, -0.046)
  line L189 (6.9311, -0.046) -> (6.9311, -3.9954)
  line L190 (6.9311, -3.9954) -> (7.7535, -3.9954)
  line L191 (7.7535, -3.9954) -> (7.7535, -4.683)
  line L192 (7.7535, -4.683) -> (6.9311, -4.683)
  line L193 (6.9311, -4.683) -> (6.9311, -6.142)
  line L194 (6.9311, -6.142) -> (6.183, -6.142)
  line L195 (6.183, -3.9954) -> (6.183, -1.2447)
  line L196 (6.183, -1.2447) -> (4.2734, -3.9954)
  line L197 (4.2734, -3.9954) -> (6.183, -3.9954)
  spline S201 degree 2 poles (8.5201, -3.1358) (8.5201, -2.0532) (8.9662, -0.7336) (9.8397, -0.0228) (10.5088, -0.0228) knots 0 0 0 1 2 3 3 3
  spline S202 degree 2 poles (10.5088, -0.0228) (10.9966, -0.0228) (11.7401, -0.4177) (12.2186, -1.1611) (12.4928, -2.2298) (12.4928, -3.1358) knots 0 0 0 1 2 3 4 4 4
  spline S203 degree 2 poles (12.4928, -3.1358) (12.4928, -4.2091) (12.0514, -5.5287) (11.1732, -6.2442) (10.5088, -6.2442) knots 0 0 0 1 2 3 3 3
  spline S204 degree 2 poles (10.5088, -6.2442) (9.626, -6.2442) (9.1242, -5.6169) knots 0 0 0 1 1 1
  spline S205 degree 2 poles (9.1242, -5.6169) (8.5201, -4.8503) (8.5201, -3.1358) knots 0 0 0 1 1 1
  spline S206 degree 2 poles (9.2914, -3.1358) (9.2914, -4.6412) (9.993, -5.6309) (10.5088, -5.6309) knots 0 0 0 1 2 2 2
  spline S207 degree 2 poles (10.5088, -5.6309) (11.0199, -5.6309) (11.7215, -4.6366) (11.7215, -3.1358) knots 0 0 0 1 2 2 2
  spline S208 degree 2 poles (11.7215, -3.1358) (11.7215, -1.6304) (11.0199, -0.6407) (10.4995, -0.6407) knots 0 0 0 1 2 2 2
  spline S209 degree 2 poles (10.4995, -0.6407) (9.9837, -0.6407) (9.6771, -1.0775) knots 0 0 0 1 1 1
  spline S210 degree 2 poles (9.6771, -1.0775) (9.2914, -1.635) (9.2914, -3.1358) knots 0 0 0 1 1 1
  spline S211 degree 2 poles (13.2548, -3.1358) (13.2548, -2.0532) (13.7008, -0.7336) (14.5743, -0.0228) (15.2434, -0.0228) knots 0 0 0 1 2 3 3 3
  spline S212 degree 2 poles (15.2434, -0.0228) (15.7313, -0.0228) (16.4747, -0.4177) (16.9533, -1.1611) (17.2274, -2.2298) (17.2274, -3.1358) knots 0 0 0 1 2 3 4 4 4
  spline S213 degree 2 poles (17.2274, -3.1358) (17.2274, -4.2091) (16.786, -5.5287) (15.9078, -6.2442) (15.2434, -6.2442) knots 0 0 0 1 2 3 3 3
  spline S214 degree 2 poles (15.2434, -6.2442) (14.3606, -6.2442) (13.8588, -5.6169) knots 0 0 0 1 1 1
  spline S215 degree 2 poles (13.8588, -5.6169) (13.2548, -4.8503) (13.2548, -3.1358) knots 0 0 0 1 1 1
  spline S216 degree 2 poles (14.0261, -3.1358) (14.0261, -4.6412) (14.7277, -5.6309) (15.2434, -5.6309) knots 0 0 0 1 2 2 2
  spline S217 degree 2 poles (15.2434, -5.6309) (15.7545, -5.6309) (16.4561, -4.6366) (16.4561, -3.1358) knots 0 0 0 1 2 2 2
  spline S218 degree 2 poles (16.4561, -3.1358) (16.4561, -1.6304) (15.7545, -0.6407) (15.2341, -0.6407) knots 0 0 0 1 2 2 2
  spline S219 degree 2 poles (15.2341, -0.6407) (14.7184, -0.6407) (14.4117, -1.0775) knots 0 0 0 1 1 1
  spline S220 degree 2 poles (14.4117, -1.0775) (14.0261, -1.635) (14.0261, -3.1358) knots 0 0 0 1 1 1
  line L198 (18.1799, -6.142) -> (18.1799, -0.046)
  line L199 (18.1799, -0.046) -> (18.928, -0.046)
  line L200 (18.928, -0.046) -> (18.928, -6.142)
  line L201 (18.928, -6.142) -> (18.1799, -6.142)
  line L202 (20.7772, -6.142) -> (20.0849, -6.142)
  line L203 (20.0849, -6.142) -> (20.0849, -0.046)
  line L204 (20.0849, -0.046) -> (20.833, -0.046)
  line L205 (20.833, -0.046) -> (20.833, -2.2205)
  spline S221 degree 2 poles (20.833, -2.2205) (21.3069, -1.6257) (22.041, -1.6257) knots 0 0 0 1 1 1
  spline S222 degree 2 poles (22.041, -1.6257) (22.4499, -1.6257) (23.1794, -1.9556) (23.6486, -2.5504) (23.9135, -3.3867) (23.9135, -3.8653) knots 0 0 0 1 2 3 4 4 4
  spline S223 degree 2 poles (23.9135, -3.8653) (23.9135, -4.999) (22.7891, -6.2396) (22.0038, -6.2396) knots 0 0 0 1 2 2 2
  spline S224 degree 2 poles (22.0038, -6.2396) (21.2232, -6.2396) (20.7772, -5.5891) knots 0 0 0 1 1 1
  line L206 (20.7772, -5.5891) -> (20.7772, -6.142)
  spline S225 degree 2 poles (20.7679, -3.8978) (20.7679, -4.6923) (20.9816, -5.0501) knots 0 0 0 1 1 1
  spline S226 degree 2 poles (20.9816, -5.0501) (21.3348, -5.6262) (21.9388, -5.6262) knots 0 0 0 1 1 1
  spline S227 degree 2 poles (21.9388, -5.6262) (22.4266, -5.6262) (23.1422, -4.7713) (23.1422, -3.9303) knots 0 0 0 1 2 2 2
  spline S228 degree 2 poles (23.1422, -3.9303) (23.1422, -3.0615) (22.4592, -2.2391) (21.9713, -2.2391) knots 0 0 0 1 2 2 2
  spline S229 degree 2 poles (21.9713, -2.2391) (21.4834, -2.2391) (20.7679, -3.094) (20.7679, -3.8978) knots 0 0 0 1 2 2 2
  line L207 (25.312, -7.9355) -> (24.7777, -7.9355)
  spline S230 degree 2 poles (24.7777, -7.9355) (26.0183, -5.9375) (26.0183, -3.9396) knots 0 0 0 1 1 1
  spline S231 degree 2 poles (26.0183, -3.9396) (26.0183, -3.159) (25.8417, -2.3877) knots 0 0 0 1 1 1
  spline S232 degree 2 poles (25.8417, -2.3877) (25.6977, -1.7651) (25.4468, -1.189) knots 0 0 0 1 1 1
  spline S233 degree 2 poles (25.4468, -1.189) (25.2841, -0.8173) (24.7777, 0.0562) knots 0 0 0 1 1 1
  line L208 (24.7777, 0.0562) -> (25.312, 0.0562)
  spline S234 degree 2 poles (25.312, 0.0562) (26.0926, -0.9892) (26.469, -2.0393) knots 0 0 0 1 1 1
  spline S235 degree 2 poles (26.469, -2.0393) (26.7896, -2.9453) (26.7896, -3.935) knots 0 0 0 1 1 1
  spline S236 degree 2 poles (26.7896, -3.935) (26.7896, -5.0594) (25.93, -7.1549) (25.312, -7.9355) knots 0 0 0 1 2 2 2
  line L209 (-17.5412, -15.7353) -> (-18.2892, -15.7353)
  line L210 (-18.2892, -15.7353) -> (-18.2892, -10.9681)
  spline S237 degree 2 poles (-18.2892, -10.9681) (-18.5587, -11.2237) (-19.4369, -11.7394) (-19.7854, -11.8695) knots 0 0 0 1 2 2 2
  line L211 (-19.7854, -11.8695) -> (-19.7854, -11.1447)
  spline S238 degree 2 poles (-19.7854, -11.1447) (-19.1581, -10.852) (-18.2195, -10.011) (-18.0244, -9.616) knots 0 0 0 1 2 2 2
  line L212 (-18.0244, -9.616) -> (-17.5412, -9.616)
  line L213 (-17.5412, -9.616) -> (-17.5412, -15.7353)
  spline S239 degree 2 poles (-15.6222, -12.7291) (-15.6222, -11.6465) (-15.1762, -10.3269) (-14.3027, -9.616) (-13.6336, -9.616) knots 0 0 0 1 2 3 3 3
  spline S240 degree 2 poles (-13.6336, -9.616) (-13.1457, -9.616) (-12.4023, -10.011) (-11.9238, -10.7544) (-11.6496, -11.8231) (-11.6496, -12.7291) knots 0 0 0 1 2 3 4 4 4
  spline S241 degree 2 poles (-11.6496, -12.7291) (-11.6496, -13.8024) (-12.091, -15.122) (-12.9692, -15.8375) (-13.6336, -15.8375) knots 0 0 0 1 2 3 3 3
  spline S242 degree 2 poles (-13.6336, -15.8375) (-14.5164, -15.8375) (-15.0182, -15.2102) knots 0 0 0 1 1 1
  spline S243 degree 2 poles (-15.0182, -15.2102) (-15.6222, -14.4436) (-15.6222, -12.7291) knots 0 0 0 1 1 1
  spline S244 degree 2 poles (-14.851, -12.7291) (-14.851, -14.2345) (-14.1494, -15.2242) (-13.6336, -15.2242) knots 0 0 0 1 2 2 2
  spline S245 degree 2 poles (-13.6336, -15.2242) (-13.1225, -15.2242) (-12.4209, -14.2299) (-12.4209, -12.7291) knots 0 0 0 1 2 2 2
  spline S246 degree 2 poles (-12.4209, -12.7291) (-12.4209, -11.2237) (-13.1225, -10.234) (-13.6429, -10.234) knots 0 0 0 1 2 2 2
  spline S247 degree 2 poles (-13.6429, -10.234) (-14.1586, -10.234) (-14.4653, -10.6708) knots 0 0 0 1 1 1
  spline S248 degree 2 poles (-14.4653, -10.6708) (-14.851, -11.2283) (-14.851, -12.7291) knots 0 0 0 1 1 1
  line L214 (-11.2407, -15.8375) -> (-9.4751, -9.5371)
  line L215 (-9.4751, -9.5371) -> (-8.8711, -9.5371)
  line L216 (-8.8711, -9.5371) -> (-10.6367, -15.8375)
  line L217 (-10.6367, -15.8375) -> (-11.2407, -15.8375)
  line L218 (-4.5918, -15.0151) -> (-4.5918, -15.7353)
  line L219 (-4.5918, -15.7353) -> (-8.6202, -15.7353)
  spline S249 degree 2 poles (-8.6202, -15.7353) (-8.6295, -15.4658) (-8.5319, -15.2149) knots 0 0 0 1 1 1
  spline S250 degree 2 poles (-8.5319, -15.2149) (-8.3786, -14.8014) (-7.7002, -14.0068) (-7.059, -13.4818) knots 0 0 0 1 2 2 2
  spline S251 degree 2 poles (-7.059, -13.4818) (-6.0694, -12.664) (-5.3724, -11.7162) (-5.3724, -11.2887) knots 0 0 0 1 2 2 2
  spline S252 degree 2 poles (-5.3724, -11.2887) (-5.3724, -10.8427) (-6.009, -10.234) (-6.5201, -10.234) knots 0 0 0 1 2 2 2
  spline S253 degree 2 poles (-6.5201, -10.234) (-7.059, -10.234) (-7.7049, -10.8845) (-7.7095, -11.456) knots 0 0 0 1 2 2 2
  line L220 (-7.7095, -11.456) -> (-8.4808, -11.377)
  spline S254 degree 2 poles (-8.4808, -11.377) (-8.4018, -10.5174) (-7.3703, -9.616) (-6.5015, -9.616) knots 0 0 0 1 2 2 2
  spline S255 degree 2 poles (-6.5015, -9.616) (-5.6233, -9.616) (-4.6011, -10.5871) (-4.6011, -11.3073) knots 0 0 0 1 2 2 2
  spline S256 degree 2 poles (-4.6011, -11.3073) (-4.6011, -11.6744) (-4.8985, -12.3806) (-5.5954, -13.1612) (-6.3993, -13.8442) knots 0 0 0 1 2 3 3 3
  spline S257 degree 2 poles (-6.3993, -13.8442) (-7.073, -14.4064) (-7.454, -14.8107) (-7.5794, -15.0151) knots 0 0 0 1 2 2 2
  line L221 (-7.5794, -15.0151) -> (-4.5918, -15.0151)
  line L222 (-3.7834, -14.1183) -> (-3.0353, -14.0208)
  spline S258 degree 2 poles (-3.0353, -14.0208) (-2.9052, -14.6573) (-2.2872, -15.2195) (-1.8412, -15.2195) knots 0 0 0 1 2 2 2
  spline S259 degree 2 poles (-1.8412, -15.2195) (-1.3115, -15.2195) (-0.5867, -14.4854) (-0.5867, -13.9464) knots 0 0 0 1 2 2 2
  spline S260 degree 2 poles (-0.5867, -13.9464) (-0.5867, -13.4307) (-1.2604, -12.7616) (-1.7808, -12.7616) knots 0 0 0 1 2 2 2
  spline S261 degree 2 poles (-1.7808, -12.7616) (-1.9899, -12.7616) (-2.3058, -12.8452) knots 0 0 0 1 1 1
  line L223 (-2.3058, -12.8452) -> (-2.2268, -12.1901)
  spline S262 degree 2 poles (-2.2268, -12.1901) (-2.1479, -12.1994) (-2.106, -12.1994) knots 0 0 0 1 1 1
  spline S263 degree 2 poles (-2.106, -12.1994) (-1.6275, -12.1994) (-0.8608, -11.6976) (-0.8608, -11.1819) knots 0 0 0 1 2 2 2
  spline S264 degree 2 poles (-0.8608, -11.1819) (-0.8608, -10.7683) (-1.4184, -10.2294) (-1.8598, -10.2294) knots 0 0 0 1 2 2 2
  spline S265 degree 2 poles (-1.8598, -10.2294) (-2.2965, -10.2294) (-2.8773, -10.7776) (-2.961, -11.3305) knots 0 0 0 1 2 2 2
  line L224 (-2.961, -11.3305) -> (-3.709, -11.1958)
  spline S266 degree 2 poles (-3.709, -11.1958) (-3.5696, -10.4431) (-2.5985, -9.616) (-1.8737, -9.616) knots 0 0 0 1 2 2 2
  spline S267 degree 2 poles (-1.8737, -9.616) (-1.3766, -9.616) (-0.5356, -10.0435) (-0.0895, -10.7823) (-0.0895, -11.1958) knots 0 0 0 1 2 3 3 3
  spline S268 degree 2 poles (-0.0895, -11.1958) (-0.0895, -11.5907) (-0.5123, -12.2412) (-0.9305, -12.4317) knots 0 0 0 1 2 2 2
  spline S269 degree 2 poles (-0.9305, -12.4317) (-0.3869, -12.5572) (0.2078, -13.3424) (0.2078, -13.9325) knots 0 0 0 1 2 2 2
  spline S270 degree 2 poles (0.2078, -13.9325) (0.2078, -14.727) (-0.9584, -15.8375) (-1.8458, -15.8375) knots 0 0 0 1 2 2 2
  spline S271 degree 2 poles (-1.8458, -15.8375) (-2.6497, -15.8375) (-3.709, -14.8803) (-3.7834, -14.1183) knots 0 0 0 1 2 2 2
  line L225 (0.5935, -15.8375) -> (2.3591, -9.5371)
  line L226 (2.3591, -9.5371) -> (2.9631, -9.5371)
  line L227 (2.9631, -9.5371) -> (1.1975, -15.8375)
  line L228 (1.1975, -15.8375) -> (0.5935, -15.8375)
  line L229 (7.2424, -15.0151) -> (7.2424, -15.7353)
  line L230 (7.2424, -15.7353) -> (3.214, -15.7353)
  spline S272 degree 2 poles (3.214, -15.7353) (3.2047, -15.4658) (3.3023, -15.2149) knots 0 0 0 1 1 1
  spline S273 degree 2 poles (3.3023, -15.2149) (3.4556, -14.8014) (4.134, -14.0068) (4.7752, -13.4818) knots 0 0 0 1 2 2 2
  spline S274 degree 2 poles (4.7752, -13.4818) (5.7649, -12.664) (6.4618, -11.7162) (6.4618, -11.2887) knots 0 0 0 1 2 2 2
  spline S275 degree 2 poles (6.4618, -11.2887) (6.4618, -10.8427) (5.8253, -10.234) (5.3142, -10.234) knots 0 0 0 1 2 2 2
  spline S276 degree 2 poles (5.3142, -10.234) (4.7752, -10.234) (4.1294, -10.8845) (4.1247, -11.456) knots 0 0 0 1 2 2 2
  line L231 (4.1247, -11.456) -> (3.3534, -11.377)
  spline S277 degree 2 poles (3.3534, -11.377) (3.4324, -10.5174) (4.4639, -9.616) (5.3328, -9.616) knots 0 0 0 1 2 2 2
  spline S278 degree 2 poles (5.3328, -9.616) (6.2109, -9.616) (7.2331, -10.5871) (7.2331, -11.3073) knots 0 0 0 1 2 2 2
  spline S279 degree 2 poles (7.2331, -11.3073) (7.2331, -11.6744) (6.9357, -12.3806) (6.2388, -13.1612) (5.435, -13.8442) knots 0 0 0 1 2 3 3 3
  spline S280 degree 2 poles (5.435, -13.8442) (4.7613, -14.4064) (4.3803, -14.8107) (4.2548, -15.0151) knots 0 0 0 1 2 2 2
  line L232 (4.2548, -15.0151) -> (7.2424, -15.0151)
  spline S281 degree 2 poles (8.0462, -12.7291) (8.0462, -11.6465) (8.4923, -10.3269) (9.3658, -9.616) (10.0349, -9.616) knots 0 0 0 1 2 3 3 3
  spline S282 degree 2 poles (10.0349, -9.616) (10.5227, -9.616) (11.2661, -10.011) (11.7447, -10.7544) (12.0188, -11.8231) (12.0188, -12.7291) knots 0 0 0 1 2 3 4 4 4
  spline S283 degree 2 poles (12.0188, -12.7291) (12.0188, -13.8024) (11.5774, -15.122) (10.6993, -15.8375) (10.0349, -15.8375) knots 0 0 0 1 2 3 3 3
  spline S284 degree 2 poles (10.0349, -15.8375) (9.152, -15.8375) (8.6502, -15.2102) knots 0 0 0 1 1 1
  spline S285 degree 2 poles (8.6502, -15.2102) (8.0462, -14.4436) (8.0462, -12.7291) knots 0 0 0 1 1 1
  spline S286 degree 2 poles (8.8175, -12.7291) (8.8175, -14.2345) (9.5191, -15.2242) (10.0349, -15.2242) knots 0 0 0 1 2 2 2
  spline S287 degree 2 poles (10.0349, -15.2242) (10.546, -15.2242) (11.2475, -14.2299) (11.2475, -12.7291) knots 0 0 0 1 2 2 2
  spline S288 degree 2 poles (11.2475, -12.7291) (11.2475, -11.2237) (10.546, -10.234) (10.0256, -10.234) knots 0 0 0 1 2 2 2
  spline S289 degree 2 poles (10.0256, -10.234) (9.5098, -10.234) (9.2032, -10.6708) knots 0 0 0 1 1 1
  spline S290 degree 2 poles (9.2032, -10.6708) (8.8175, -11.2283) (8.8175, -12.7291) knots 0 0 0 1 1 1
  line L233 (16.7116, -15.0151) -> (16.7116, -15.7353)
  line L234 (16.7116, -15.7353) -> (12.6833, -15.7353)
  spline S291 degree 2 poles (12.6833, -15.7353) (12.674, -15.4658) (12.7715, -15.2149) knots 0 0 0 1 1 1
  spline S292 degree 2 poles (12.7715, -15.2149) (12.9249, -14.8014) (13.6032, -14.0068) (14.2444, -13.4818) knots 0 0 0 1 2 2 2
  spline S293 degree 2 poles (14.2444, -13.4818) (15.2341, -12.664) (15.9311, -11.7162) (15.9311, -11.2887) knots 0 0 0 1 2 2 2
  spline S294 degree 2 poles (15.9311, -11.2887) (15.9311, -10.8427) (15.2945, -10.234) (14.7834, -10.234) knots 0 0 0 1 2 2 2
  spline S295 degree 2 poles (14.7834, -10.234) (14.2444, -10.234) (13.5986, -10.8845) (13.594, -11.456) knots 0 0 0 1 2 2 2
  line L235 (13.594, -11.456) -> (12.8227, -11.377)
  spline S296 degree 2 poles (12.8227, -11.377) (12.9016, -10.5174) (13.9331, -9.616) (14.802, -9.616) knots 0 0 0 1 2 2 2
  spline S297 degree 2 poles (14.802, -9.616) (15.6802, -9.616) (16.7024, -10.5871) (16.7024, -11.3073) knots 0 0 0 1 2 2 2
  spline S298 degree 2 poles (16.7024, -11.3073) (16.7024, -11.6744) (16.405, -12.3806) (15.708, -13.1612) (14.9042, -13.8442) knots 0 0 0 1 2 3 3 3
  spline S299 degree 2 poles (14.9042, -13.8442) (14.2305, -14.4064) (13.8495, -14.8107) (13.724, -15.0151) knots 0 0 0 1 2 2 2
  line L236 (13.724, -15.0151) -> (16.7116, -15.0151)
  line L237 (17.5155, -14.1369) -> (18.3007, -14.0719)
  spline S300 degree 2 poles (18.3007, -14.0719) (18.389, -14.648) (19.0209, -15.2242) (19.4716, -15.2242) knots 0 0 0 1 2 2 2
  spline S301 degree 2 poles (19.4716, -15.2242) (20.0198, -15.2242) (20.7633, -14.4064) (20.7633, -13.7327) knots 0 0 0 1 2 2 2
  spline S302 degree 2 poles (20.7633, -13.7327) (20.7633, -13.0915) (20.0477, -12.3481) (19.4623, -12.3481) knots 0 0 0 1 2 2 2
  spline S303 degree 2 poles (19.4623, -12.3481) (19.0999, -12.3481) (18.5191, -12.678) (18.3518, -12.9428) knots 0 0 0 1 2 2 2
  line L238 (18.3518, -12.9428) -> (17.6502, -12.8499)